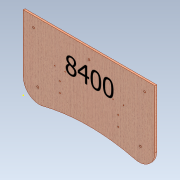
# Autodesk Inventor part: FTC Outside Panels
Saved by Autodesk Inventor 2020 (Build 240168000, 168)
## iProperties
Created: 2022-09-23
Part Number: FTC Outside Panels
Material: Wood (Oak)
Document SubType Name: Modeling
Designer: Jason
Density: 0.76 g/cm^3
Appearance: White Oak - Natural Medium Gloss
Mass: 371.39 g
Surface Area: 1832.51 cm^2
Volume: 488.671 cm^3
Author: Allan
Autodesk Inventor part; units mm, degrees
ref_plane "YZ Plane" through (0, 0, 0) normal (1, 0, 0) x (0, 1, 0)
ref_plane "XZ Plane" through (0, 0, 0) normal (0, 1, 0) x (-1, 0, 0)
ref_plane "XY Plane" through (0, 0, 0) normal (0, 0, 1) x (1, 0, 0)
sketch "Sketch1" plane through (0, 0, 0) normal (0, 0, 1) x (1, 0, 0)
  line L0 (49.2125, 0) -> (54.6328, 0)
  line L1 (357.1875, 0) -> (350.9902, 0)
  arc A0 (0, 49.2125) -> (65.0875, 2.6308) centre (49.2125, 49.2125) ccw
  arc A1 (345.2239, 1.4763) -> (406.4, 49.2125) centre (357.1875, 49.2125) ccw
  arc A2 (203.2, 19.05) -> (54.6328, 0) centre (202.8115, -566.7686) ccw
  arc A3 (350.9902, 0) -> (345.2239, 1.4763) centre (202.8115, -566.7686) ccw
  arc A4 (65.0875, 2.6308) -> (54.6328, 0) centre (202.8115, -566.7686) ccw
  arc A5 (350.9902, 0) -> (203.2, 19.05) centre (202.8115, -566.7686) ccw
  line L2 (0, 49.2125) -> (0, 228.6)
  line L3 (406.4, 228.6) -> (406.4, 49.2125)
  line L4 (0, 228.6) -> (406.4, 228.6)
  point P0 (0, 0)
  point P1 (57.0671, 0.6309)
  constraints: 16 point on circle, 10 end point, 6 centre point, 1 perpendicular, 1 vertical
extrude "Extrusion1" add sketch "Sketch1" along normal blind 5.5563 contours A0 L2 L4 L3 A1 A5 A2
sketch "Sketch5" plane through (0, 0, 5.5563) normal (0, 0, 1) x (1, 0, 0)
  line L0 (128.7512, 178.3406) -> (279.9627, 178.3406) construction
  line L1 (279.9627, 178.3406) -> (279.9627, 123.3225) construction
  line L2 (279.9627, 123.3225) -> (128.7512, 123.3225) construction
  line L3 (128.7512, 123.3225) -> (128.7512, 178.3406) construction
  point P0 (0, 0)
  constraints: 2 other
sketch "Sketch6" plane through (0, 0, 5.5563) normal (0, 0, 1) x (1, 0, 0)
  line L0 (406.4, 228.6) -> (0, 228.6)
  line L1 (0, 228.6) -> (0, 49.2125)
  circle A0 centre (31.75, 196.85) radius 2.9337
  line L2 (406.4, 49.2125) -> (406.4, 228.6)
  circle A1 centre (374.65, 196.85) radius 2.9337
  circle A2 centre (203.2, 196.85) radius 2.9337
  arc A3 (345.2239, 1.4763) -> (406.4, 49.2125) centre (357.1875, 49.2125) ccw
  circle A4 centre (361.7391, 44.6609) radius 2.9337
  arc A5 (0, 49.2125) -> (57.0671, 0.6309) centre (49.2125, 49.2125) ccw
  circle A6 centre (44.6609, 44.6609) radius 2.9337
  point P0 (0, 0)
  point P1 (0, 0)
  constraints: 7 centre point, 6 end point, 4 point on circle
extrude "Extrusion6" cut sketch "Sketch6" against normal up to surface (5.5563 mm away)
sketch "Sketch7" plane through (0, 0, 5.5563) normal (0, 0, 1) x (1, 0, 0)
  ellipse E0 centre (293.3334, 94.2801) end of major axis (293.3295, 96.2801) minor radius 2
  ellipse E1 centre (293.3643, 62.2802) end of major axis (293.3569, 64.2802) minor radius 2
  circle A0 centre (361.7412, 44.6631) radius 2.9337
  line L0 (361.7412, 44.6631) -> (293.3643, 44.6631)
  line L1 (293.3643, 44.6631) -> (293.3643, 62.2802)
  ellipse E2 centre (113.007, 94.278) end of major axis (113.0032, 96.278) minor radius 2
  ellipse E3 centre (113.0379, 62.2781) end of major axis (113.0305, 64.2781) minor radius 2
  line L2 (113.0379, 44.6609) -> (113.0379, 62.2781)
  circle A1 centre (293.3643, 78.2802) radius 4.699
  circle A2 centre (113.0379, 78.278) radius 4.699
  circle A3 centre (44.6609, 44.6609) radius 2.9337
  line L3 (44.6609, 44.6609) -> (113.0379, 44.6609)
  point P0 (0, 0)
  point P1 (0, 0)
  dimension "d59" = 17.6171
  dimension "d60" = 68.3769
  dimension "d61" = 17.6171
  dimension "d62" = 9.398
  dimension "d63" = 9.398
  dimension "d64" = 68.3769
  constraints: 8 end point, 4 centre point, 2 horizontal, 1 perpendicular, 1 vertical, 8 other
  measures "d59" distance of L0.end L1.end
  measures "d60" distance of L0.start L0.end
  measures "d61" distance of L2.start L2.end
  measures "d62" diameter of A1
  measures "d63" diameter of A2
  measures "d64" distance of L3.start L2.start
extrude "Extrusion7" cut sketch "Sketch7" against normal through all contours E0 | E1 | E2 | E3
sketch "Sketch8" plane through (0, 0, 5.5563) normal (0, 0, 1) x (1, 0, 0)
  ellipse E0 centre (309.3078, 127.6497) end of major axis (309.3104, 126.2971) minor radius 1.3525
  ellipse E1 centre (277.3079, 127.5882) end of major axis (277.3105, 126.2356) minor radius 1.3525
  ellipse E2 centre (293.3334, 94.2801) end of major axis (293.3295, 96.2801) minor radius 2
  ellipse E3 centre (293.3334, 94.2801) end of major axis (293.3295, 96.2801) minor radius 2 projected
  ellipse E4 centre (128.9815, 127.6475) end of major axis (128.9841, 126.295) minor radius 1.3525
  ellipse E5 centre (96.9816, 127.586) end of major axis (96.9842, 126.2335) minor radius 1.3525
  ellipse E6 centre (113.007, 94.278) end of major axis (113.0032, 96.278) minor radius 2
  ellipse E7 centre (113.007, 94.278) end of major axis (113.0032, 96.278) minor radius 2 projected
  point P0 (0, 0)
  constraints: 4 centre point, 6 other
extrude "Extrusion8" cut sketch "Sketch8" against normal through all contours E0 | E1 | E4 | E5
body "Solid1"
